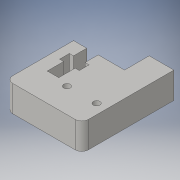
# Autodesk Inventor part: A8-0018
Saved by Autodesk Inventor 2016 SP2 (Build 200236200, 236)
## iProperties
Created: 2017-04-22
Part Number: A8-0018
Material: Generic
Document SubType Name: Modeling
Designer: EV
Density: 1 g/cm^3
Appearance: Default
Author: EV
Autodesk Inventor part; units mm, degrees
ref_plane "YZ Plane" through (0, 0, 0) normal (1, 0, 0) x (0, 1, 0)
sketch "Sketch1" plane through (0, 0, 0) normal (0, 1, 0) x (-1, 0, 0)
  line L0 (0, 0) -> (23, 0)
  line L1 (23, 0) -> (23, -20.5)
  line L2 (7.5, -28) -> (0, -28)
  line L3 (0, -28) -> (0, 0)
  line L4 (7.5, -28) -> (7.5, -20.5)
  line L5 (7.5, -20.5) -> (23, -20.5)
  line L6 (19, -20.5) -> (19, -16.5)
  line L7 (19, -16.5) -> (20.25, -16.5)
  line L8 (20.25, -16.5) -> (20.25, -13.5)
  line L9 (20.25, -13.5) -> (19, -13.5)
  line L10 (19, -13.5) -> (19, -8.5)
  line L11 (19, -8.5) -> (15.5, -8.5)
  line L12 (15.5, -8.5) -> (15.5, -13.5)
  line L13 (15.5, -13.5) -> (14.25, -13.5)
  line L14 (14.25, -13.5) -> (14.25, -16.5)
  line L15 (14.25, -16.5) -> (15.5, -16.5)
  line L16 (15.5, -20.5) -> (15.5, -16.5)
  line L17 (17.25, -8.5) -> (17.25, -20.5) construction
  dimension "d0" = 28
  dimension "d1" = 23
  dimension "d2" = 7.5
  dimension "d3" = 20.5
  dimension "d4" = 3.5
  dimension "d5" = 6
  dimension "d6" = 4
  dimension "d7" = 3
  dimension "d8" = 5
  dimension "d9" = 4
  constraints: 36 end point, 11 perpendicular, 10 point on line, 2 parallel, 2 vertical, 1 collinear, 1 horizontal, 1 midpoint
  measures "d0" distance of L2.end L0.start
  measures "d1" distance between parallel lines of L3 L1
  measures "d2" distance of L2.start L2.end
  measures "d3" distance of L0.end L1.end
  measures "d4" distance between parallel lines of L16 L6
  measures "d5" distance between parallel lines of L14 L8
  measures "d6" distance of L16.start L15.end
  measures "d7" distance of L13.end L14.end
  measures "d8" distance of L11.end L12.end
  measures "d9" distance between parallel lines of L1 L6
extrude "Extrusion1" add sketch "Sketch1" along normal blind 8 contours L0 L1 L5 L6 L7 L8 L9 L10 L11 L12 L13 L14 L15 L16 L4 L2 L3
sketch "Sketch2" plane through (0, 8, 0) normal (0, 1, 0) x (1, 0, 0)
  line L0 (0, 0) -> (0, 28) construction
  line L1 (0, 28) -> (-7.5, 28) construction
  line L2 (-7.5, 28) -> (-7.5, 20.5) construction
  line L3 (-7.5, 20.5) -> (-15.5, 20.5) construction
  line L4 (-15.5, 20.5) -> (-15.5, 16.5) construction
  line L5 (-15.5, 16.5) -> (-14.25, 16.5) construction
  line L6 (-14.25, 16.5) -> (-14.25, 13.5) construction
  line L7 (-14.25, 13.5) -> (-15.5, 13.5) construction
  line L8 (-15.5, 13.5) -> (-15.5, 8.5) construction
  line L9 (-15.5, 8.5) -> (-19, 8.5) construction
  line L10 (-19, 8.5) -> (-19, 13.5) construction
  line L11 (-19, 13.5) -> (-20.25, 13.5) construction
  line L12 (-20.25, 13.5) -> (-20.25, 16.5) construction
  line L13 (-20.25, 16.5) -> (-19, 16.5) construction
  line L14 (-19, 16.5) -> (-19, 20.5) construction
  line L15 (-19, 20.5) -> (-23, 20.5) construction
  line L16 (-23, 20.5) -> (-23, 0) construction
  line L17 (-23, 0) -> (0, 0) construction
  point P0 (-12, 7.5)
  point P1 (-3, 7.5)
  dimension "d12" = 7.5
  dimension "d13" = 3
  dimension "d14" = 9
  constraints: 1 horizontal alignment
  measures "d12" distance from line of L17 point (-3, 7.5)
  measures "d13" distance from line of L0 point (-3, 7.5)
  measures "d14" distance of point (-3, 7.5) point (-12, 7.5)
hole "Hole1" at (-12, 8, -7.5) at (-3, 8, -7.5) direction (0, -1, 0) diameter 2 end through all
fillet "Fillet1" radius 2 2 edges at (-23, 4, 0) (0, 4, 0)
ref_plane "Work Plane1" through (0, 4, 0) normal (0, 1, 0) x (-1, 0, 0)
ref_plane "Work Plane2" through (-17.25, 0, -8.5) normal (1, 0, 0) x (0, 0, -1)
equation "\"d23\" = 0.5 * THICKNESS"
equation "\"THICKNESS\" = 8"
body "Solid1"
